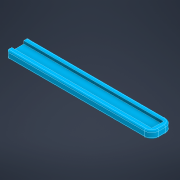
# Autodesk Inventor part: ArmRestCushion
Saved by Autodesk Inventor 2021 (Build 250183000, 183)
## iProperties
Created: 2021-01-30
Part Number: ArmRestCushion
Material: Generic
Document SubType Name: Modeling
Designer: argon
Density: 1 g/cm^3
Appearance: Sky Blue Medium
Author: argon
Autodesk Inventor part; units mm, degrees
ref_plane "YZ Plane" through (0, 0, 0) normal (1, 0, 0) x (0, 1, 0)
ref_plane "XZ Plane" through (0, 0, 0) normal (0, 1, 0) x (-1, 0, 0)
ref_plane "XY Plane" through (0, 0, 0) normal (0, 0, 1) x (1, 0, 0)
sketch "Sketch1" plane through (0, 0, 0) normal (0, 1, 0) x (-1, 0, 0)
  line L0 (233.18, 20) -> (-233.18, 20)
  line L1 (-233.18, 20) -> (-233.18, -20)
  line L2 (-233.18, -20) -> (233.18, -20)
  line L3 (233.18, -20) -> (233.18, 20)
  line L4 (233.18, 20) -> (-233.18, -20) construction
  line L5 (-233.18, 20) -> (233.18, -20) construction
  line L6 (233.18, 35) -> (-248.18, 35)
  line L7 (-248.18, 35) -> (-248.18, -35)
  line L8 (-248.18, -35) -> (233.18, -35)
  line L9 (233.18, -35) -> (233.18, 35)
  line L10 (233.18, 35) -> (-248.18, -35) construction
  line L11 (-248.18, 35) -> (233.18, -35) construction
  point P0 (0, 0)
  point P1 (-7.5, 0)
  dimension "d0" = 466.36
  dimension "d1" = 40
  dimension "d2" = 15
  dimension "d3" = 15
  constraints: 24 end point, 4 midpoint, 4 parallel, 2 horizontal, 2 perpendicular, 1 collinear, 1 horizontal alignment
  measures "d0" distance of L0.start L0.end
  measures "d1" distance of L2.end L0.start
  measures "d2" distance between parallel lines of L7 L1
  measures "d3" distance between parallel lines of L2 L8
extrude "Extrusion1" add sketch "Sketch1" along normal blind 15 contours L3 L2 L1 L0
extrude "Extrusion2" add sketch "Sketch1" along normal blind 25 contours L0 L1 L2 L9 L8 L7 L6
fillet "Fillet1" radius 24 2 edges at (248.18, 12.5, -35) (248.18, 12.5, 35)
fillet "Fillet2" radius 5 13 edges at (241.1506, 0, -27.9706) (248.18, 0, 0) (241.1506, 0, 27.9706) (-4.5, 0, 35) (-4.5, 0, -35) (-233.18, 12.5, -35) (-233.18, 12.5, 35) (241.1506, 25, -27.9706) (248.18, 25, 0) (241.1506, 25, 27.9706) (-4.5, 25, 35) (-4.5, 25, -35) (-233.18, 0, 0)
body "Solid1"
